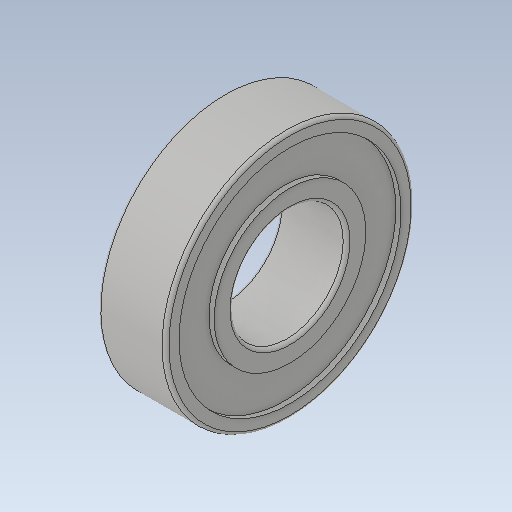
# Autodesk Inventor part: bearing_6900
Saved by Autodesk Inventor 2020.2 (Build 242310000, 310)
## iProperties
Created: 2022-11-04
Part Number: bearing_6900
Material: Generic
Catalog Web Link: www.cadenas.de
Description: 6000_bearing-Deep Groove Ball Bearings
Vendor: MISUMI
Document SubType Name: Modeling
Designer: psAdmin
Manufacturer: MISUMI
Mass: 1.66105 g
Surface Area: 12.7379 cm^2
Volume: 1.66105 cm^3
Density: 1 g/cm^3
Appearance: PSOLRGB-175-175-175
Category: PARTsolutions
Company: MISUMI
PSOL_IDENT_0: {$CADENAS_DATA/23d-libs/misumi/metric/accessories/bearing_6000.prj},170 {VTYP=3D},{NB=bearing_6900},
PSOL_IDENT_1: {LINA=bearing_6900},{NN=6000_bearing},{DATE=30.06.2021 13:30:08},{GEOMDATE=24.10.2013 00:00:00},{VER
PSOL_IDENT_2: SION=},{LINEID=30},{WBVAR=},{WBNUMERIC=}  {NB=bearing_6900},{LINA=bearing_6900},{KT=DUMMY},{PN=beari
PSOL_IDENT_3: ng_6900},{BN=6900},{DD=10},{D=22},{B=6},{RR=0.3},{DSMIN=12.0},{DS1=13.00},{DSMAX=13.00},{DDHH=20.0},
PSOL_IDENT_4: {R=0.3},{R1=0.200},{R2=0.300},{MASS=9},{MASS11=9},{AA=5.1000},{BB=1.2000},{CC=1.7000},{DD1=20.800}
NB: bearing_6900
NN: 6000_bearing
NT: Deep Groove Ball Bearings
NBSYN: $PN.
LINA: bearing_6900
CATALOG: Misumi
PN: bearing_6900
BN: 6900
DD: 10
D: 22
B: 6
RR: 0.3
DSMIN: 12
DDHH: 20
R: 0.3
MASS11: 9
SUPPLIER: MISUMI
ARTICLENO: bearing_6900
BOMINFO: bearing_6900
CREATOR: CADENAS GmbH
Title: bearing_6900
Author: Cadenas PARTsolutions
Comments: Deep Groove Ball Bearings
Autodesk Inventor part; units mm, degrees
sketch "Sketch_1" plane through (0, 0, 0) normal (0, 0, 1) x (1, 0, 0)
  line L0 (6, 0) -> (0, 0)
  arc A0 (0, 5.3) -> (0.3, 5) centre (0.3, 5.3) ccw
  line L1 (0.3, 5) -> (5.7, 5)
  arc A1 (5.7, 5) -> (6, 5.3) centre (5.7, 5.3) ccw
  line L2 (6, 5.3) -> (6, 6.7)
  line L3 (6, 6.7) -> (5.55, 6.7)
  line L4 (5.55, 6.7) -> (5.55, 9.8)
  line L5 (5.55, 9.8) -> (6, 9.8)
  line L6 (6, 9.8) -> (6, 10.7)
  arc A2 (6, 10.7) -> (5.7, 11) centre (5.7, 10.7) ccw
  line L7 (5.7, 11) -> (0.3, 11)
  arc A3 (0.3, 11) -> (0, 10.7) centre (0.3, 10.7) ccw
  line L8 (0, 10.7) -> (0, 9.8)
  line L9 (0, 9.8) -> (0.45, 9.8)
  line L10 (0.45, 9.8) -> (0.45, 6.7)
  line L11 (0.45, 6.7) -> (0, 6.7)
  line L12 (0, 6.7) -> (0, 5.3)
  constraints: 26 end point, 8 point on circle, 4 centre point
revolve "Revolution1" add sketch "Sketch_1" angle 360 about axis through (6, 0, 0) along (1, 0, 0)
ref_plane "center_point_XY" through (3, 0, 0) normal (1, 0, 0) x (0, 0, -1)
ref_plane "center_point_YZ" through (3, 0, 0) normal (0, 0, -1) x (0, 1, 0)
ref_plane "center_point_ZX" through (3, 0, 0) normal (0, 1, 0) x (1, 0, 0)
ref_plane "to_housing_XY" through (0, 0, 0) normal (1, 0, 0) x (0, 0, -1)
ref_plane "to_housing_YZ" through (0, 0, 0) normal (0, 0, -1) x (0, 1, 0)
ref_plane "to_housing_ZX" through (0, 0, 0) normal (0, 1, 0) x (1, 0, 0)
ref_plane "to_ring_XY" through (5.1, 0, 0) normal (1, 0, 0) x (0, 0, -1)
ref_plane "to_ring_YZ" through (5.1, 0, 0) normal (0, 0, -1) x (0, 1, 0)
ref_plane "to_ring_ZX" through (5.1, 0, 0) normal (0, 1, 0) x (1, 0, 0)
body "Solid1"
